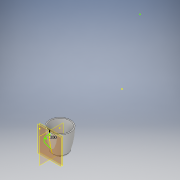
# Autodesk Inventor part: Mug
Saved by Autodesk Inventor 2017 (Build 210142000, 142)
## iProperties
Created: 2018-03-16
Part Number: Mug
Material: Generic
Document SubType Name: Modeling
Designer: landontracy
Density: 1 g/cm^3
Appearance: Default
Author: landontracy
Autodesk Inventor part; units mm, degrees
ref_plane "XZ Plane" through (0, 0, 0) normal (0, 1, 0) x (-1, 0, 0)
sketch "Mug outline" plane through (0, 0, 0) normal (0, 0, 1) x (1, 0, 0)
  arc A0 (-4.453, 8.7954) -> (10.5231, -89.6417) centre (351.0022, 12.5162) ccw
  arc A1 (0.6313, 8.7954) -> (17.373, -88.6665) centre (310.2491, 11.8115) ccw
  line L0 (-4.453, 8.7954) -> (0.6313, 8.7954)
  line L1 (23.7564, -102.9497) -> (34.9669, -102.9497)
  arc A2 (17.373, -88.6665) -> (19.9041, -93.4241) centre (32.3151, -83.7692) ccw
  arc A3 (10.5231, -89.6417) -> (22.0313, -102.752) centre (30.3393, -83.8531) ccw
  arc A4 (22.0313, -102.752) -> (23.7564, -102.9497) centre (23.4424, -98.0659) ccw
  arc A5 (19.9041, -93.4241) -> (23.6525, -95.479) centre (24.886, -88.7827) ccw
  line L2 (23.6525, -95.479) -> (34.9669, -95.479)
  line L3 (34.9669, -95.479) -> (47.3988, -95.479)
  line L4 (34.9669, -102.9497) -> (47.3988, -102.9497)
  line L5 (47.3988, -95.479) -> (47.3988, -102.9497)
  line L6 (47.3988, -108.675) -> (47.3988, 3.3674)
  point P0 (0, 0)
  constraints: 14 end point, 12 point on circle, 6 centre point, 4 horizontal, 2 vertical, 1 point on line
revolve "Revolution1" add sketch "Mug outline" angle 360 about axis through (47.3988, -108.675, 0) along (0, 1, 0)
ref_plane "Work Plane1" through (0, 0, 50.8) normal (0, 0, 1) x (1, 0, 0)
ref_plane "Work Plane2" through (0, 0, 42.8625) normal (0, 0, 1) x (1, 0, 0)
sketch "Sketch2" plane through (0, 0, 50.8) normal (0, 0, 1) x (1, 0, 0)
  point P0 (0, 0)
sketch "Sketch3" plane through (0, 0, 50.8) normal (0, 0, 1) x (1, 0, 0)
  circle A0 centre (47.0902, 0) radius 3.81
  point P0 (0, 0)
  dimension "d5" = 7.62
  constraints: 1 centre point
  measures "d5" diameter of A0
ref_plane "Work Plane3" through (46.0375, 0, 0) normal (1, 0, 0) x (0, 1, 0)
sketch "Sketch4" plane through (46.0375, 0, 0) normal (1, 0, 0) x (0, 1, 0)
  point P0 (0, 0)
sketch "Sketch5" plane through (46.0375, 0, 0) normal (1, 0, 0) x (0, 1, 0)
  line L0 (0.4364, 51.1257) -> (0.4364, 65.491)
  arc A0 (0.4364, 65.491) -> (-5.0303, 76.1087) centre (-12.608, 65.491) ccw
  arc A1 (-9.7447, 77.6675) -> (-25.4206, 73.0631) centre (-10.2573, 50.426) ccw
  arc A2 (8.7954, 51.8518) -> (-89.6417, 36.8757) centre (12.5162, -303.6034) ccw projected
  arc A3 (-25.4206, 73.0631) -> (-66.0724, 43.0752) centre (284.5102, -389.63) ccw
  arc A4 (-5.0303, 76.1087) -> (-9.7447, 77.6675) centre (-9.9025, 69.2819) ccw
  point P0 (0, 0)
  constraints: 9 point on circle, 4 centre point, 4 tangent, 2 end point, 1 vertical
body "Solid1"
